Autodesk Fusion 360 part; units mm, degrees
note: some values were not read from the file. Set by a fixed rule: which sketch regions a step uses.
(part 13 of 59)
  spline S70 degree 5 poles (-29.0307, 13.4213) (-29.0307, 13.4213) (-29.0309, 13.4213) (-29.0313, 13.4213) (-29.0318, 13.4213) (-29.0325, 13.4213) (-29.0334, 13.4213) (-29.0344, 13.4214) (-29.0355, 13.4214) (-29.0367, 13.4214) (-29.038, 13.4214) (-29.0394, 13.4214) (-29.0409, 13.4214) (-29.0425, 13.4214) (-29.0443, 13.4214) (-29.0461, 13.4214) (-29.0481, 13.4214) (-29.0501, 13.4214) (-29.0522, 13.4214) (-29.0545, 13.4214) (-29.0568, 13.4214) (-29.0592, 13.4213) (-29.0618, 13.4213) (-29.0644, 13.4212) (-29.0671, 13.4212) (-29.0699, 13.4211) (-29.0728, 13.4211) (-29.0758, 13.421) (-29.0788, 13.4209) (-29.082, 13.4208) (-29.0852, 13.4208) (-29.0886, 13.4206) (-29.092, 13.4205) (-29.0955, 13.4204) (-29.0991, 13.4203) (-29.1028, 13.4201) (-29.1065, 13.42) (-29.1103, 13.4198) (-29.1143, 13.4197) (-29.1183, 13.4195) (-29.1223, 13.4193) (-29.1265, 13.4191) (-29.1307, 13.4189) (-29.135, 13.4186) (-29.1394, 13.4184) (-29.1439, 13.4182) (-29.1484, 13.4179) (-29.153, 13.4176) (-29.1577, 13.4173) (-29.1624, 13.417) (-29.1673, 13.4167) (-29.1722, 13.4164) (-29.1771, 13.4161) (-29.1822, 13.4157) (-29.1873, 13.4153) (-29.1925, 13.415) (-29.1977, 13.4146) (-29.203, 13.4141) (-29.2084, 13.4137) (-29.2139, 13.4133) (-29.2194, 13.4128) (-29.225, 13.4124) (-29.2306, 13.4119) (-29.2363, 13.4114) (-29.2421, 13.4109) (-29.248, 13.4103) (-29.2539, 13.4098) (-29.2599, 13.4092) (-29.2659, 13.4087) (-29.272, 13.4081) (-29.2781, 13.4075) (-29.2844, 13.4068) (-29.2906, 13.4062) (-29.297, 13.4055) (-29.3034, 13.4049) (-29.3099, 13.4042) (-29.3164, 13.4035) (-29.323, 13.4027) (-29.3296, 13.402) (-29.3363, 13.4012) (-29.343, 13.4005) (-29.3498, 13.3997) (-29.3567, 13.3989) (-29.3636, 13.398) (-29.3706, 13.3972) (-29.3777, 13.3963) (-29.3847, 13.3954) (-29.3919, 13.3945) (-29.3991, 13.3936) (-29.4063, 13.3927) (-29.4137, 13.3917) (-29.421, 13.3907) (-29.4284, 13.3897) (-29.4359, 13.3887) (-29.4434, 13.3877) (-29.451, 13.3866) (-29.4586, 13.3856) (-29.4663, 13.3845) (-29.474, 13.3834) (-29.4818, 13.3822) (-29.4896, 13.3811) (-29.4975, 13.3799) (-29.5054, 13.3787) (-29.5134, 13.3775) (-29.5214, 13.3763) (-29.5295, 13.375) (-29.5376, 13.3738) (-29.5458, 13.3725) (-29.554, 13.3712) (-29.5623, 13.3698) (-29.5706, 13.3685) (-29.5789, 13.3671) (-29.5873, 13.3657) (-29.5958, 13.3643) (-29.6043, 13.3629) (-29.6128, 13.3614) (-29.6214, 13.36) (-29.6301, 13.3585) (-29.6388, 13.3569) (-29.6475, 13.3554) (-29.6563, 13.3538) (-29.6651, 13.3523) (-29.6739, 13.3507) (-29.6828, 13.349) (-29.6918, 13.3474) (-29.7008, 13.3457) (-29.7098, 13.344) (-29.7189, 13.3423) (-29.728, 13.3406) (-29.7372, 13.3388) (-29.7464, 13.3371) (-29.7556, 13.3353) (-29.7649, 13.3334) (-29.7742, 13.3316) (-29.7836, 13.3297) (-29.793, 13.3279) (-29.8025, 13.3259) (-29.812, 13.324) (-29.8215, 13.3221) (-29.8311, 13.3201) (-29.8407, 13.3181) (-29.8503, 13.3161) (-29.86, 13.314) (-29.8697, 13.312) (-29.8795, 13.3099) (-29.8893, 13.3078) (-29.8992, 13.3056) (-29.909, 13.3035) (-29.919, 13.3013) (-29.9289, 13.2991) (-29.9389, 13.2969) (-29.949, 13.2946) (-29.959, 13.2923) (-29.9691, 13.29) (-29.9793, 13.2877) (-29.9895, 13.2854) (-29.9997, 13.283) (-30.0099, 13.2806) (-30.0202, 13.2782) (-30.0306, 13.2758) (-30.0409, 13.2733) (-30.0513, 13.2708) (-30.0618, 13.2683) (-30.0722, 13.2658) (-30.0827, 13.2632) (-30.0933, 13.2606) (-30.1038, 13.258) (-30.1145, 13.2554) (-30.1251, 13.2528) (-30.1358, 13.2501) (-30.1465, 13.2474) (-30.1572, 13.2447) (-30.168, 13.2419) (-30.1788, 13.2391) (-30.1897, 13.2364) (-30.2005, 13.2335) (-30.2114, 13.2307) (-30.2224, 13.2278) (-30.2334, 13.2249) (-30.2444, 13.222) (-30.2554, 13.2191) (-30.2665, 13.2161) (-30.2776, 13.2131) (-30.2887, 13.2101) (-30.2999, 13.2071) (-30.3111, 13.204) (-30.3223, 13.2009) (-30.3336, 13.1978) (-30.3448, 13.1947) (-30.3562, 13.1915) (-30.3675, 13.1883) (-30.3789, 13.1851) (-30.3903, 13.1819) (-30.4017, 13.1786) (-30.4132, 13.1753) (-30.4247, 13.172) (-30.4362, 13.1687) (-30.4478, 13.1653) (-30.4594, 13.1619) (-30.471, 13.1585) (-30.4827, 13.1551) (-30.4943, 13.1516) (-30.506, 13.1481) (-30.5178, 13.1446) (-30.5295, 13.1411) (-30.5413, 13.1375) (-30.5531, 13.1339) (-30.565, 13.1303) (-30.5769, 13.1267) (-30.5888, 13.123) (-30.6007, 13.1193) (-30.6126, 13.1156) (-30.6246, 13.1118) (-30.6366, 13.1081) (-30.6487, 13.1043) (-30.6607, 13.1005) (-30.6728, 13.0966) (-30.685, 13.0927) (-30.6971, 13.0889) (-30.7093, 13.0849) (-30.7215, 13.081) (-30.7337, 13.077) (-30.7459, 13.073) (-30.7582, 13.069) (-30.7705, 13.0649) (-30.7828, 13.0609) (-30.7952, 13.0568) (-30.8076, 13.0526) (-30.82, 13.0485) (-30.8324, 13.0443) (-30.8448, 13.0401) (-30.8573, 13.0359) (-30.8698, 13.0316) (-30.8823, 13.0273) (-30.8949, 13.023) (-30.9075, 13.0187) (-30.9201, 13.0143) (-30.9327, 13.0099) (-30.9453, 13.0055) (-30.958, 13.0011) (-30.9707, 12.9966) (-30.9809, 12.993) (-30.9885, 12.9903) (-30.9936, 12.9885) (-30.9962, 12.9876) knots 0 0 0 0 0 0 0.00416667 0.00833333 0.0125 0.01666667 0.02083333 0.025 0.02916667 0.03333333 0.0375 0.04166667 0.04583333 0.05 0.05416667 0.05833333 0.0625 0.06666667 0.07083333 0.075 0.07916667 0.08333333 0.0875 0.09166667 0.09583333 0.1 0.10416667 0.10833333 0.1125 0.11666667 0.12083333 0.125 0.12916667 0.13333333 0.1375 0.14166667 0.14583333 0.15 0.15416667 0.15833333 0.1625 0.16666667 0.17083333 0.175 0.17916667 0.18333333 0.1875 0.19166667 0.19583333 0.2 0.20416667 0.20833333 0.2125 0.21666667 0.22083333 0.225 0.22916667 0.23333333 0.2375 0.24166667 0.24583333 0.25 0.25416667 0.25833333 0.2625 0.26666667 0.27083333 0.275 0.27916667 0.28333333 0.2875 0.29166667 0.29583333 0.3 0.30416667 0.30833333 0.3125 0.31666667 0.32083333 0.325 0.32916667 0.33333333 0.3375 0.34166667 0.34583333 0.35 0.35416667 0.35833333 0.3625 0.36666667 0.37083333 0.375 0.37916667 0.38333333 0.3875 0.39166667 0.39583333 0.4 0.40416667 0.40833333 0.4125 0.41666667 0.42083333 0.425 0.42916667 0.43333333 0.4375 0.44166667 0.44583333 0.45 0.45416667 0.45833333 0.4625 0.46666667 0.47083333 0.475 0.47916667 0.48333333 0.4875 0.49166667 0.49583333 0.5 0.50416667 0.50833333 0.5125 0.51666667 0.52083333 0.525 0.52916667 0.53333333 0.5375 0.54166667 0.54583333 0.55 0.55416667 0.55833333 0.5625 0.56666667 0.57083333 0.575 0.57916667 0.58333333 0.5875 0.59166667 0.59583333 0.6 0.60416667 0.60833333 0.6125 0.61666667 0.62083333 0.625 0.62916667 0.63333333 0.6375 0.64166667 0.64583333 0.65 0.65416667 0.65833333 0.6625 0.66666667 0.67083333 0.675 0.67916667 0.68333333 0.6875 0.69166667 0.69583333 0.7 0.70416667 0.70833333 0.7125 0.71666667 0.72083333 0.725 0.72916667 0.73333333 0.7375 0.74166667 0.74583333 0.75 0.75416667 0.75833333 0.7625 0.76666667 0.77083333 0.775 0.77916667 0.78333333 0.7875 0.79166667 0.79583333 0.8 0.80416667 0.80833333 0.8125 0.81666667 0.82083333 0.825 0.82916667 0.83333333 0.8375 0.84166667 0.84583333 0.85 0.85416667 0.85833333 0.8625 0.86666667 0.87083333 0.875 0.87916667 0.88333333 0.8875 0.89166667 0.89583333 0.9 0.90416667 0.90833333 0.9125 0.91666667 0.92083333 0.925 0.92916667 0.93333333 0.9375 0.94166667 0.94583333 0.95 0.95416667 0.95833333 0.9625 0.96666667 0.97083333 0.975 0.97916667 0.98333333 0.9875 0.99166667 0.99583333 1 1 1 1 1 1
  spline S71 degree 5 poles (15.3132, 37.1806) (15.3132, 37.1807) (15.3133, 37.1809) (15.3135, 37.1812) (15.3138, 37.1816) (15.3142, 37.1822) (15.3146, 37.183) (15.3151, 37.1838) (15.3157, 37.1848) (15.3163, 37.1858) (15.3169, 37.1869) (15.3177, 37.1881) (15.3184, 37.1895) (15.3193, 37.1909) (15.3201, 37.1924) (15.321, 37.194) (15.322, 37.1956) (15.323, 37.1974) (15.3241, 37.1993) (15.3252, 37.2012) (15.3263, 37.2033) (15.3275, 37.2054) (15.3287, 37.2076) (15.33, 37.2099) (15.3313, 37.2122) (15.3327, 37.2147) (15.3341, 37.2172) (15.3355, 37.2198) (15.337, 37.2225) (15.3385, 37.2253) (15.34, 37.2282) (15.3416, 37.2311) (15.3432, 37.2341) (15.3449, 37.2372) (15.3465, 37.2404) (15.3482, 37.2437) (15.35, 37.247) (15.3518, 37.2504) (15.3536, 37.2539) (15.3554, 37.2574) (15.3573, 37.261) (15.3592, 37.2647) (15.3611, 37.2685) (15.3631, 37.2723) (15.3651, 37.2763) (15.3671, 37.2802) (15.3691, 37.2843) (15.3712, 37.2884) (15.3733, 37.2926) (15.3754, 37.2969) (15.3775, 37.3012) (15.3797, 37.3056) (15.3819, 37.3101) (15.3841, 37.3147) (15.3863, 37.3193) (15.3886, 37.3239) (15.3909, 37.3287) (15.3932, 37.3335) (15.3955, 37.3384) (15.3979, 37.3433) (15.4002, 37.3483) (15.4026, 37.3534) (15.405, 37.3585) (15.4075, 37.3637) (15.4099, 37.369) (15.4124, 37.3743) (15.4149, 37.3797) (15.4174, 37.3852) (15.4199, 37.3907) (15.4224, 37.3962) (15.425, 37.4019) (15.4275, 37.4076) (15.4301, 37.4133) (15.4327, 37.4192) (15.4353, 37.425) (15.438, 37.431) (15.4406, 37.437) (15.4433, 37.443) (15.446, 37.4492) (15.4486, 37.4553) (15.4514, 37.4616) (15.4541, 37.4679) (15.4568, 37.4742) (15.4595, 37.4806) (15.4623, 37.4871) (15.4651, 37.4936) (15.4678, 37.5002) (15.4706, 37.5069) (15.4734, 37.5136) (15.4762, 37.5203) (15.4791, 37.5271) (15.4819, 37.534) (15.4848, 37.5409) (15.4876, 37.5479) (15.4905, 37.5549) (15.4933, 37.562) (15.4962, 37.5691) (15.4991, 37.5763) (15.502, 37.5836) (15.5049, 37.5909) (15.5078, 37.5982) (15.5108, 37.6056) (15.5137, 37.6131) (15.5166, 37.6206) (15.5196, 37.6282) (15.5226, 37.6358) (15.5255, 37.6434) (15.5285, 37.6512) (15.5315, 37.6589) (15.5344, 37.6668) (15.5374, 37.6746) (15.5404, 37.6826) (15.5434, 37.6905) (15.5464, 37.6986) (15.5494, 37.7066) (15.5524, 37.7148) (15.5555, 37.7229) (15.5585, 37.7312) (15.5615, 37.7394) (15.5645, 37.7478) (15.5676, 37.7562) (15.5706, 37.7646) (15.5737, 37.7731) (15.5767, 37.7816) (15.5798, 37.7901) (15.5828, 37.7988) (15.5859, 37.8074) (15.5889, 37.8161) (15.592, 37.8249) (15.595, 37.8337) (15.5981, 37.8426) (15.6012, 37.8515) (15.6042, 37.8604) (15.6073, 37.8694) (15.6104, 37.8785) (15.6134, 37.8876) (15.6165, 37.8967) (15.6196, 37.9059) (15.6227, 37.9151) (15.6257, 37.9244) (15.6288, 37.9337) (15.6319, 37.9431) (15.635, 37.9525) (15.638, 37.962) (15.6411, 37.9715) (15.6442, 37.981) (15.6473, 37.9906) (15.6503, 38.0003) (15.6534, 38.0099) (15.6565, 38.0197) (15.6596, 38.0294) (15.6626, 38.0393) (15.6657, 38.0491) (15.6688, 38.059) (15.6718, 38.069) (15.6749, 38.079) (15.6779, 38.089) (15.681, 38.0991) (15.6841, 38.1092) (15.6871, 38.1194) (15.6902, 38.1296) (15.6932, 38.1398) (15.6963, 38.1501) (15.6993, 38.1604) (15.7023, 38.1708) (15.7054, 38.1812) (15.7084, 38.1917) (15.7114, 38.2022) (15.7145, 38.2127) (15.7175, 38.2233) (15.7205, 38.2339) (15.7235, 38.2446) (15.7265, 38.2553) (15.7295, 38.266) (15.7325, 38.2768) (15.7355, 38.2877) (15.7385, 38.2985) (15.7415, 38.3094) (15.7445, 38.3204) (15.7475, 38.3314) (15.7504, 38.3424) (15.7534, 38.3535) (15.7564, 38.3646) (15.7593, 38.3757) (15.7623, 38.3869) (15.7652, 38.3982) (15.7682, 38.4094) (15.7711, 38.4207) (15.774, 38.4321) (15.7769, 38.4435) (15.7798, 38.4549) (15.7828, 38.4663) (15.7857, 38.4778) (15.7886, 38.4894) (15.7914, 38.501) (15.7943, 38.5126) (15.7972, 38.5242) (15.8001, 38.5359) (15.8029, 38.5477) (15.8058, 38.5594) (15.8086, 38.5712) (15.8115, 38.5831) (15.8143, 38.595) (15.8171, 38.6069) (15.8199, 38.6188) (15.8227, 38.6308) (15.8255, 38.6428) (15.8283, 38.6549) (15.8311, 38.667) (15.8339, 38.6792) (15.8367, 38.6913) (15.8394, 38.7035) (15.8422, 38.7158) (15.8449, 38.7281) (15.8477, 38.7404) (15.8504, 38.7528) (15.8531, 38.7651) (15.8558, 38.7776) (15.8585, 38.79) (15.8612, 38.8025) (15.8639, 38.8151) (15.8666, 38.8276) (15.8692, 38.8403) (15.8719, 38.8529) (15.8745, 38.8656) (15.8771, 38.8783) (15.8798, 38.891) (15.8824, 38.9038) (15.885, 38.9166) (15.8876, 38.9295) (15.8902, 38.9424) (15.8927, 38.9553) (15.8953, 38.9682) (15.8979, 38.9812) (15.9004, 38.9943) (15.9029, 39.0073) (15.9055, 39.0204) (15.908, 39.0335) (15.9105, 39.0467) (15.913, 39.0599) (15.9154, 39.0731) (15.9174, 39.0837) (15.9189, 39.0917) (15.9199, 39.097) (15.9204, 39.0997) knots 0 0 0 0 0 0 0.00416667 0.00833333 0.0125 0.01666667 0.02083333 0.025 0.02916667 0.03333333 0.0375 0.04166667 0.04583333 0.05 0.05416667 0.05833333 0.0625 0.06666667 0.07083333 0.075 0.07916667 0.08333333 0.0875 0.09166667 0.09583333 0.1 0.10416667 0.10833333 0.1125 0.11666667 0.12083333 0.125 0.12916667 0.13333333 0.1375 0.14166667 0.14583333 0.15 0.15416667 0.15833333 0.1625 0.16666667 0.17083333 0.175 0.17916667 0.18333333 0.1875 0.19166667 0.19583333 0.2 0.20416667 0.20833333 0.2125 0.21666667 0.22083333 0.225 0.22916667 0.23333333 0.2375 0.24166667 0.24583333 0.25 0.25416667 0.25833333 0.2625 0.26666667 0.27083333 0.275 0.27916667 0.28333333 0.2875 0.29166667 0.29583333 0.3 0.30416667 0.30833333 0.3125 0.31666667 0.32083333 0.325 0.32916667 0.33333333 0.3375 0.34166667 0.34583333 0.35 0.35416667 0.35833333 0.3625 0.36666667 0.37083333 0.375 0.37916667 0.38333333 0.3875 0.39166667 0.39583333 0.4 0.40416667 0.40833333 0.4125 0.41666667 0.42083333 0.425 0.42916667 0.43333333 0.4375 0.44166667 0.44583333 0.45 0.45416667 0.45833333 0.4625 0.46666667 0.47083333 0.475 0.47916667 0.48333333 0.4875 0.49166667 0.49583333 0.5 0.50416667 0.50833333 0.5125 0.51666667 0.52083333 0.525 0.52916667 0.53333333 0.5375 0.54166667 0.54583333 0.55 0.55416667 0.55833333 0.5625 0.56666667 0.57083333 0.575 0.57916667 0.58333333 0.5875 0.59166667 0.59583333 0.6 0.60416667 0.60833333 0.6125 0.61666667 0.62083333 0.625 0.62916667 0.63333333 0.6375 0.64166667 0.64583333 0.65 0.65416667 0.65833333 0.6625 0.66666667 0.67083333 0.675 0.67916667 0.68333333 0.6875 0.69166667 0.69583333 0.7 0.70416667 0.70833333 0.7125 0.71666667 0.72083333 0.725 0.72916667 0.73333333 0.7375 0.74166667 0.74583333 0.75 0.75416667 0.75833333 0.7625 0.76666667 0.77083333 0.775 0.77916667 0.78333333 0.7875 0.79166667 0.79583333 0.8 0.80416667 0.80833333 0.8125 0.81666667 0.82083333 0.825 0.82916667 0.83333333 0.8375 0.84166667 0.84583333 0.85 0.85416667 0.85833333 0.8625 0.86666667 0.87083333 0.875 0.87916667 0.88333333 0.8875 0.89166667 0.89583333 0.9 0.90416667 0.90833333 0.9125 0.91666667 0.92083333 0.925 0.92916667 0.93333333 0.9375 0.94166667 0.94583333 0.95 0.95416667 0.95833333 0.9625 0.96666667 0.97083333 0.975 0.97916667 0.98333333 0.9875 0.99166667 0.99583333 1 1 1 1 1 1
  line L155 (29.0298, 11.5787) -> (29.0307, 11.5787)
  arc A82 (26.6221, 1.6453) -> (27.0473, 2.7529) centre (0, 12.5) ccw
  spline S72 degree 5 poles (28.5878, 17.6346) (28.5879, 17.6347) (28.5881, 17.6347) (28.5884, 17.6348) (28.5889, 17.6349) (28.5896, 17.635) (28.5905, 17.6352) (28.5915, 17.6354) (28.5925, 17.6356) (28.5937, 17.6358) (28.595, 17.6361) (28.5964, 17.6363) (28.5979, 17.6367) (28.5995, 17.637) (28.6012, 17.6374) (28.603, 17.6377) (28.6049, 17.6381) (28.6069, 17.6386) (28.6089, 17.639) (28.6111, 17.6395) (28.6134, 17.64) (28.6158, 17.6406) (28.6182, 17.6411) (28.6208, 17.6417) (28.6234, 17.6423) (28.6262, 17.643) (28.629, 17.6436) (28.6319, 17.6443) (28.6349, 17.645) (28.6379, 17.6458) (28.6411, 17.6465) (28.6443, 17.6473) (28.6477, 17.6481) (28.6511, 17.649) (28.6545, 17.6499) (28.6581, 17.6508) (28.6617, 17.6517) (28.6655, 17.6527) (28.6693, 17.6536) (28.6731, 17.6546) (28.6771, 17.6557) (28.6811, 17.6567) (28.6852, 17.6578) (28.6893, 17.6589) (28.6936, 17.6601) (28.6979, 17.6613) (28.7023, 17.6625) (28.7067, 17.6637) (28.7112, 17.6649) (28.7158, 17.6662) (28.7205, 17.6675) (28.7252, 17.6689) (28.73, 17.6702) (28.7349, 17.6716) (28.7398, 17.673) (28.7448, 17.6745) (28.7498, 17.676) (28.7549, 17.6775) (28.7601, 17.679) (28.7654, 17.6806) (28.7707, 17.6822) (28.776, 17.6838) (28.7815, 17.6854) (28.7869, 17.6871) (28.7925, 17.6888) (28.7981, 17.6905) (28.8038, 17.6923) (28.8095, 17.6941) (28.8153, 17.6959) (28.8211, 17.6978) (28.827, 17.6996) (28.833, 17.7015) (28.839, 17.7035) (28.8451, 17.7054) (28.8512, 17.7074) (28.8573, 17.7094) (28.8636, 17.7115) (28.8699, 17.7136) (28.8762, 17.7157) (28.8826, 17.7178) (28.889, 17.72) (28.8955, 17.7222) (28.9021, 17.7244) (28.9087, 17.7266) (28.9153, 17.7289) (28.922, 17.7312) (28.9288, 17.7336) (28.9356, 17.7359) (28.9424, 17.7383) (28.9493, 17.7408) (28.9563, 17.7432) (28.9633, 17.7457) (28.9703, 17.7482) (28.9774, 17.7508) (28.9846, 17.7533) (28.9918, 17.7559) (28.999, 17.7586) (29.0063, 17.7612) (29.0136, 17.7639) (29.021, 17.7666) (29.0284, 17.7694) (29.0358, 17.7722) (29.0433, 17.775) (29.0509, 17.7778) (29.0585, 17.7807) (29.0661, 17.7836) (29.0738, 17.7865) (29.0815, 17.7895) (29.0893, 17.7925) (29.0971, 17.7955) (29.105, 17.7986) (29.1129, 17.8016) (29.1208, 17.8047) (29.1288, 17.8079) (29.1368, 17.8111) (29.1448, 17.8143) (29.1529, 17.8175) (29.1611, 17.8207) (29.1692, 17.824) (29.1775, 17.8273) (29.1857, 17.8307) (29.194, 17.8341) (29.2023, 17.8375) (29.2107, 17.8409) (29.2191, 17.8444) (29.2276, 17.8479) (29.2361, 17.8514) (29.2446, 17.855) (29.2531, 17.8586) (29.2617, 17.8622) (29.2704, 17.8658) (29.279, 17.8695) (29.2878, 17.8732) (29.2965, 17.877) (29.3053, 17.8807) (29.3141, 17.8846) (29.3229, 17.8884) (29.3318, 17.8922) (29.3407, 17.8961) (29.3497, 17.9001) (29.3587, 17.904) (29.3677, 17.908) (29.3767, 17.912) (29.3858, 17.9161) (29.395, 17.9201) (29.4041, 17.9242) (29.4133, 17.9284) (29.4225, 17.9325) (29.4318, 17.9367) (29.441, 17.941) (29.4504, 17.9452) (29.4597, 17.9495) (29.4691, 17.9538) (29.4785, 17.9582) (29.4879, 17.9625) (29.4974, 17.967) (29.5069, 17.9714) (29.5165, 17.9759) (29.526, 17.9804) (29.5356, 17.9849) (29.5452, 17.9895) (29.5549, 17.994) (29.5646, 17.9987) (29.5743, 18.0033) (29.584, 18.008) (29.5938, 18.0127) (29.6036, 18.0175) (29.6134, 18.0222) (29.6233, 18.027) (29.6332, 18.0319) (29.6431, 18.0367) (29.653, 18.0416) (29.663, 18.0466) (29.673, 18.0515) (29.683, 18.0565) (29.6931, 18.0615) (29.7032, 18.0666) (29.7133, 18.0717) (29.7234, 18.0768) (29.7336, 18.0819) (29.7437, 18.0871) (29.754, 18.0923) (29.7642, 18.0975) (29.7745, 18.1028) (29.7847, 18.1081) (29.7951, 18.1134) (29.8054, 18.1188) (29.8158, 18.1242) (29.8262, 18.1296) (29.8366, 18.135) (29.847, 18.1405) (29.8575, 18.146) (29.868, 18.1515) (29.8785, 18.1571) (29.889, 18.1627) (29.8996, 18.1683) (29.9102, 18.174) (29.9208, 18.1797) (29.9314, 18.1854) (29.9421, 18.1912) (29.9527, 18.197) (29.9634, 18.2028) (29.9742, 18.2086) (29.9849, 18.2145) (29.9957, 18.2204) (30.0065, 18.2263) (30.0173, 18.2323) (30.0281, 18.2383) (30.039, 18.2443) (30.0499, 18.2504) (30.0608, 18.2565) (30.0717, 18.2626) (30.0826, 18.2688) (30.0936, 18.2749) (30.1046, 18.2811) (30.1156, 18.2874) (30.1266, 18.2937) (30.1377, 18.3) (30.1487, 18.3063) (30.1598, 18.3127) (30.1709, 18.3191) (30.1821, 18.3255) (30.1932, 18.3319) (30.2044, 18.3384) (30.2156, 18.3449) (30.2268, 18.3515) (30.238, 18.3581) (30.2492, 18.3647) (30.2605, 18.3713) (30.2718, 18.378) (30.2831, 18.3847) (30.2944, 18.3914) (30.3058, 18.3982) (30.3171, 18.405) (30.3285, 18.4118) (30.3399, 18.4187) (30.3513, 18.4255) (30.3628, 18.4325) (30.3742, 18.4394) (30.3857, 18.4464) (30.3972, 18.4534) (30.4064, 18.459) (30.4133, 18.4633) (30.4179, 18.4661) (30.4202, 18.4675) knots 0 0 0 0 0 0 0.00416667 0.00833333 0.0125 0.01666667 0.02083333 0.025 0.02916667 0.03333333 0.0375 0.04166667 0.04583333 0.05 0.05416667 0.05833333 0.0625 0.06666667 0.07083333 0.075 0.07916667 0.08333333 0.0875 0.09166667 0.09583333 0.1 0.10416667 0.10833333 0.1125 0.11666667 0.12083333 0.125 0.12916667 0.13333333 0.1375 0.14166667 0.14583333 0.15 0.15416667 0.15833333 0.1625 0.16666667 0.17083333 0.175 0.17916667 0.18333333 0.1875 0.19166667 0.19583333 0.2 0.20416667 0.20833333 0.2125 0.21666667 0.22083333 0.225 0.22916667 0.23333333 0.2375 0.24166667 0.24583333 0.25 0.25416667 0.25833333 0.2625 0.26666667 0.27083333 0.275 0.27916667 0.28333333 0.2875 0.29166667 0.29583333 0.3 0.30416667 0.30833333 0.3125 0.31666667 0.32083333 0.325 0.32916667 0.33333333 0.3375 0.34166667 0.34583333 0.35 0.35416667 0.35833333 0.3625 0.36666667 0.37083333 0.375 0.37916667 0.38333333 0.3875 0.39166667 0.39583333 0.4 0.40416667 0.40833333 0.4125 0.41666667 0.42083333 0.425 0.42916667 0.43333333 0.4375 0.44166667 0.44583333 0.45 0.45416667 0.45833333 0.4625 0.46666667 0.47083333 0.475 0.47916667 0.48333333 0.4875 0.49166667 0.49583333 0.5 0.50416667 0.50833333 0.5125 0.51666667 0.52083333 0.525 0.52916667 0.53333333 0.5375 0.54166667 0.54583333 0.55 0.55416667 0.55833333 0.5625 0.56666667 0.57083333 0.575 0.57916667 0.58333333 0.5875 0.59166667 0.59583333 0.6 0.60416667 0.60833333 0.6125 0.61666667 0.62083333 0.625 0.62916667 0.63333333 0.6375 0.64166667 0.64583333 0.65 0.65416667 0.65833333 0.6625 0.66666667 0.67083333 0.675 0.67916667 0.68333333 0.6875 0.69166667 0.69583333 0.7 0.70416667 0.70833333 0.7125 0.71666667 0.72083333 0.725 0.72916667 0.73333333 0.7375 0.74166667 0.74583333 0.75 0.75416667 0.75833333 0.7625 0.76666667 0.77083333 0.775 0.77916667 0.78333333 0.7875 0.79166667 0.79583333 0.8 0.80416667 0.80833333 0.8125 0.81666667 0.82083333 0.825 0.82916667 0.83333333 0.8375 0.84166667 0.84583333 0.85 0.85416667 0.85833333 0.8625 0.86666667 0.87083333 0.875 0.87916667 0.88333333 0.8875 0.89166667 0.89583333 0.9 0.90416667 0.90833333 0.9125 0.91666667 0.92083333 0.925 0.92916667 0.93333333 0.9375 0.94166667 0.94583333 0.95 0.95416667 0.95833333 0.9625 0.96666667 0.97083333 0.975 0.97916667 0.98333333 0.9875 0.99166667 0.99583333 1 1 1 1 1 1
  line L156 (28.9679, 10.3817) -> (28.9671, 10.3818)
  line L157 (2.0967, -16.1734) -> (2.1182, -16.4671)
  arc A83 (28.1181, -0.5527) -> (28.5147, 0.3382) centre (0, 12.5) ccw
  spline S73 degree 5 poles (2.755, 43.3773) (2.7539, 43.3749) (2.7515, 43.37) (2.748, 43.3627) (2.7434, 43.353) (2.7376, 43.3408) (2.7319, 43.3287) (2.7262, 43.3165) (2.7205, 43.3044) (2.7149, 43.2924) (2.7092, 43.2803) (2.7036, 43.2683) (2.6981, 43.2563) (2.6925, 43.2443) (2.687, 43.2323) (2.6815, 43.2204) (2.6761, 43.2085) (2.6707, 43.1966) (2.6653, 43.1847) (2.6599, 43.1728) (2.6545, 43.161) (2.6492, 43.1492) (2.6439, 43.1374) (2.6387, 43.1256) (2.6335, 43.1139) (2.6283, 43.1022) (2.6231, 43.0905) (2.6179, 43.0788) (2.6128, 43.0672) (2.6077, 43.0555) (2.6027, 43.0439) (2.5977, 43.0324) (2.5927, 43.0208) (2.5877, 43.0093) (2.5827, 42.9978) (2.5778, 42.9863) (2.5729, 42.9749) (2.5681, 42.9634) (2.5632, 42.952) (2.5584, 42.9407) (2.5537, 42.9293) (2.5489, 42.918) (2.5442, 42.9067) (2.5395, 42.8954) (2.5348, 42.8841) (2.5302, 42.8729) (2.5256, 42.8617) (2.521, 42.8506) (2.5165, 42.8394) (2.5119, 42.8283) (2.5074, 42.8172) (2.503, 42.8061) (2.4985, 42.7951) (2.4941, 42.7841) (2.4897, 42.7731) (2.4854, 42.7621) (2.481, 42.7512) (2.4767, 42.7403) (2.4725, 42.7294) (2.4682, 42.7186) (2.464, 42.7078) (2.4598, 42.697) (2.4557, 42.6862) (2.4515, 42.6755) (2.4474, 42.6648) (2.4433, 42.6541) (2.4393, 42.6435) (2.4353, 42.6329) (2.4313, 42.6223) (2.4273, 42.6118) (2.4234, 42.6012) (2.4194, 42.5907) (2.4156, 42.5803) (2.4117, 42.5699) (2.4079, 42.5595) (2.4041, 42.5491) (2.4003, 42.5388) (2.3965, 42.5284) (2.3928, 42.5182) (2.3891, 42.5079) (2.3855, 42.4977) (2.3818, 42.4875) (2.3782, 42.4774) (2.3746, 42.4673) (2.3711, 42.4572) (2.3675, 42.4471) (2.364, 42.4371) (2.3606, 42.4271) (2.3571, 42.4172) (2.3537, 42.4073) (2.3503, 42.3974) (2.3469, 42.3875) (2.3436, 42.3777) (2.3403, 42.368) (2.337, 42.3582) (2.3337, 42.3485) (2.3305, 42.3388) (2.3273, 42.3292) (2.3241, 42.3196) (2.321, 42.31) (2.3178, 42.3005) (2.3147, 42.291) (2.3117, 42.2815) (2.3086, 42.2721) (2.3056, 42.2627) (2.3026, 42.2534) (2.2996, 42.2441) (2.2967, 42.2348) (2.2938, 42.2255) (2.2909, 42.2163) (2.288, 42.2072) (2.2852, 42.1981) (2.2824, 42.189) (2.2796, 42.1799) (2.2769, 42.1709) (2.2741, 42.1619) (2.2714, 42.153) (2.2688, 42.1441) (2.2661, 42.1353) (2.2635, 42.1265) (2.2609, 42.1177) (2.2583, 42.109) (2.2558, 42.1003) (2.2533, 42.0917) (2.2508, 42.083) (2.2483, 42.0745) (2.2458, 42.066) (2.2434, 42.0575) (2.241, 42.0491) (2.2387, 42.0407) (2.2363, 42.0323) (2.234, 42.024) (2.2317, 42.0158) (2.2295, 42.0075) (2.2272, 41.9994) (2.225, 41.9912) (2.2228, 41.9832) (2.2207, 41.9751) (2.2185, 41.9671) (2.2164, 41.9592) (2.2143, 41.9513) (2.2123, 41.9434) (2.2102, 41.9356) (2.2082, 41.9279) (2.2062, 41.9202) (2.2043, 41.9125) (2.2023, 41.9049) (2.2004, 41.8973) (2.1985, 41.8898) (2.1967, 41.8823) (2.1948, 41.8749) (2.193, 41.8675) (2.1912, 41.8602) (2.1895, 41.8529) (2.1877, 41.8457) (2.186, 41.8386) (2.1843, 41.8314) (2.1827, 41.8244) (2.181, 41.8174) (2.1794, 41.8104) (2.1778, 41.8035) (2.1762, 41.7967) (2.1747, 41.7899) (2.1731, 41.7831) (2.1716, 41.7764) (2.1702, 41.7698) (2.1687, 41.7632) (2.1673, 41.7567) (2.1659, 41.7502) (2.1645, 41.7438) (2.1631, 41.7374) (2.1618, 41.7311) (2.1605, 41.7249) (2.1592, 41.7187) (2.1579, 41.7126) (2.1567, 41.7065) (2.1554, 41.7005) (2.1542, 41.6946) (2.153, 41.6887) (2.1519, 41.6829) (2.1507, 41.6771) (2.1496, 41.6714) (2.1485, 41.6658) (2.1475, 41.6602) (2.1464, 41.6547) (2.1454, 41.6493) (2.1444, 41.6439) (2.1434, 41.6386) (2.1424, 41.6334) (2.1415, 41.6282) (2.1406, 41.6231) (2.1397, 41.618) (2.1388, 41.6131) (2.138, 41.6081) (2.1371, 41.6033) (2.1363, 41.5985) (2.1355, 41.5938) (2.1347, 41.5892) (2.134, 41.5847) (2.1332, 41.5802) (2.1325, 41.5758) (2.1318, 41.5714) (2.1312, 41.5672) (2.1305, 41.563) (2.1299, 41.5589) (2.1292, 41.5549) (2.1286, 41.5509) (2.1281, 41.547) (2.1275, 41.5432) (2.127, 41.5395) (2.1264, 41.5359) (2.1259, 41.5323) (2.1254, 41.5289) (2.125, 41.5255) (2.1245, 41.5222) (2.1241, 41.5189) (2.1237, 41.5158) (2.1233, 41.5128) (2.1229, 41.5098) (2.1225, 41.5069) (2.1222, 41.5041) (2.1219, 41.5015) (2.1215, 41.4989) (2.1212, 41.4963) (2.121, 41.4939) (2.1207, 41.4916) (2.1204, 41.4894) (2.1202, 41.4873) (2.12, 41.4852) (2.1198, 41.4833) (2.1196, 41.4815) (2.1194, 41.4798) (2.1192, 41.4781) (2.1191, 41.4766) (2.1189, 41.4752) (2.1188, 41.4739) (2.1187, 41.4727) (2.1186, 41.4716) (2.1185, 41.4706) (2.1184, 41.4698) (2.1184, 41.469) (2.1183, 41.4685) (2.1183, 41.4682) (2.1183, 41.468) (2.1183, 41.4679) knots -1 -1 -1 -1 -1 -1 -0.99583333 -0.99166667 -0.9875 -0.98333333 -0.97916667 -0.975 -0.97083333 -0.96666667 -0.9625 -0.95833333 -0.95416667 -0.95 -0.94583333 -0.94166667 -0.9375 -0.93333333 -0.92916667 -0.925 -0.92083333 -0.91666667 -0.9125 -0.90833333 -0.90416667 -0.9 -0.89583333 -0.89166667 -0.8875 -0.88333333 -0.87916667 -0.875 -0.87083333 -0.86666667 -0.8625 -0.85833333 -0.85416667 -0.85 -0.84583333 -0.84166667 -0.8375 -0.83333333 -0.82916667 -0.825 -0.82083333 -0.81666667 -0.8125 -0.80833333 -0.80416667 -0.8 -0.79583333 -0.79166667 -0.7875 -0.78333333 -0.77916667 -0.775 -0.77083333 -0.76666667 -0.7625 -0.75833333 -0.75416667 -0.75 -0.74583333 -0.74166667 -0.7375 -0.73333333 -0.72916667 -0.725 -0.72083333 -0.71666667 -0.7125 -0.70833333 -0.70416667 -0.7 -0.69583333 -0.69166667 -0.6875 -0.68333333 -0.67916667 -0.675 -0.67083333 -0.66666667 -0.6625 -0.65833333 -0.65416667 -0.65 -0.64583333 -0.64166667 -0.6375 -0.63333333 -0.62916667 -0.625 -0.62083333 -0.61666667 -0.6125 -0.60833333 -0.60416667 -0.6 -0.59583333 -0.59166667 -0.5875 -0.58333333 -0.57916667 -0.575 -0.57083333 -0.56666667 -0.5625 -0.55833333 -0.55416667 -0.55 -0.54583333 -0.54166667 -0.5375 -0.53333333 -0.52916667 -0.525 -0.52083333 -0.51666667 -0.5125 -0.50833333 -0.50416667 -0.5 -0.49583333 -0.49166667 -0.4875 -0.48333333 -0.47916667 -0.475 -0.47083333 -0.46666667 -0.4625 -0.45833333 -0.45416667 -0.45 -0.44583333 -0.44166667 -0.4375 -0.43333333 -0.42916667 -0.425 -0.42083333 -0.41666667 -0.4125 -0.40833333 -0.40416667 -0.4 -0.39583333 -0.39166667 -0.3875 -0.38333333 -0.37916667 -0.375 -0.37083333 -0.36666667 -0.3625 -0.35833333 -0.35416667 -0.35 -0.34583333 -0.34166667 -0.3375 -0.33333333 -0.32916667 -0.325 -0.32083333 -0.31666667 -0.3125 -0.30833333 -0.30416667 -0.3 -0.29583333 -0.29166667 -0.2875 -0.28333333 -0.27916667 -0.275 -0.27083333 -0.26666667 -0.2625 -0.25833333 -0.25416667 -0.25 -0.24583333 -0.24166667 -0.2375 -0.23333333 -0.22916667 -0.225 -0.22083333 -0.21666667 -0.2125 -0.20833333 -0.20416667 -0.2 -0.19583333 -0.19166667 -0.1875 -0.18333333 -0.17916667 -0.175 -0.17083333 -0.16666667 -0.1625 -0.15833333 -0.15416667 -0.15 -0.14583333 -0.14166667 -0.1375 -0.13333333 -0.12916667 -0.125 -0.12083333 -0.11666667 -0.1125 -0.10833333 -0.10416667 -0.1 -0.09583333 -0.09166667 -0.0875 -0.08333333 -0.07916667 -0.075 -0.07083333 -0.06666667 -0.0625 -0.05833333 -0.05416667 -0.05 -0.04583333 -0.04166667 -0.0375 -0.03333333 -0.02916667 -0.025 -0.02083333 -0.01666667 -0.0125 -0.00833333 -0.00416667 0 0 0 0 0 0
  spline S74 degree 5 poles (24.6806, -2.8132) (24.6807, -2.8132) (24.6809, -2.8133) (24.6812, -2.8135) (24.6816, -2.8138) (24.6822, -2.8142) (24.683, -2.8146) (24.6838, -2.8151) (24.6848, -2.8157) (24.6858, -2.8163) (24.6869, -2.8169) (24.6881, -2.8177) (24.6895, -2.8184) (24.6909, -2.8193) (24.6924, -2.8201) (24.694, -2.821) (24.6956, -2.822) (24.6974, -2.823) (24.6993, -2.8241) (24.7012, -2.8252) (24.7033, -2.8263) (24.7054, -2.8275) (24.7076, -2.8287) (24.7099, -2.83) (24.7122, -2.8313) (24.7147, -2.8327) (24.7172, -2.8341) (24.7198, -2.8355) (24.7225, -2.837) (24.7253, -2.8385) (24.7282, -2.84) (24.7311, -2.8416) (24.7341, -2.8432) (24.7372, -2.8449) (24.7404, -2.8465) (24.7437, -2.8482) (24.747, -2.85) (24.7504, -2.8518) (24.7539, -2.8536) (24.7574, -2.8554) (24.761, -2.8573) (24.7647, -2.8592) (24.7685, -2.8611) (24.7723, -2.8631) (24.7763, -2.8651) (24.7802, -2.8671) (24.7843, -2.8691) (24.7884, -2.8712) (24.7926, -2.8733) (24.7969, -2.8754) (24.8012, -2.8775) (24.8056, -2.8797) (24.8101, -2.8819) (24.8147, -2.8841) (24.8193, -2.8863) (24.8239, -2.8886) (24.8287, -2.8909) (24.8335, -2.8932) (24.8384, -2.8955) (24.8433, -2.8979) (24.8483, -2.9002) (24.8534, -2.9026) (24.8585, -2.905) (24.8637, -2.9075) (24.869, -2.9099) (24.8743, -2.9124) (24.8797, -2.9149) (24.8852, -2.9174) (24.8907, -2.9199) (24.8962, -2.9224) (24.9019, -2.925) (24.9076, -2.9275) (24.9133, -2.9301) (24.9192, -2.9327) (24.925, -2.9353) (24.931, -2.938) (24.937, -2.9406) (24.943, -2.9433) (24.9492, -2.946) (24.9553, -2.9486) (24.9616, -2.9514) (24.9679, -2.9541) (24.9742, -2.9568) (24.9806, -2.9595) (24.9871, -2.9623) (24.9936, -2.9651) (25.0002, -2.9678) (25.0069, -2.9706) (25.0136, -2.9734) (25.0203, -2.9762) (25.0271, -2.9791) (25.034, -2.9819) (25.0409, -2.9848) (25.0479, -2.9876) (25.0549, -2.9905) (25.062, -2.9933) (25.0691, -2.9962) (25.0763, -2.9991) (25.0836, -3.002) (25.0909, -3.0049) (25.0982, -3.0078) (25.1056, -3.0108) (25.1131, -3.0137) (25.1206, -3.0166) (25.1282, -3.0196) (25.1358, -3.0226) (25.1434, -3.0255) (25.1512, -3.0285) (25.1589, -3.0315) (25.1668, -3.0344) (25.1746, -3.0374) (25.1826, -3.0404) (25.1905, -3.0434) (25.1986, -3.0464) (25.2066, -3.0494) (25.2148, -3.0524) (25.2229, -3.0555) (25.2312, -3.0585) (25.2394, -3.0615) (25.2478, -3.0645) (25.2562, -3.0676) (25.2646, -3.0706) (25.2731, -3.0737) (25.2816, -3.0767) (25.2901, -3.0798) (25.2988, -3.0828) (25.3074, -3.0859) (25.3161, -3.0889) (25.3249, -3.092) (25.3337, -3.095) (25.3426, -3.0981) (25.3515, -3.1012) (25.3604, -3.1042) (25.3694, -3.1073) (25.3785, -3.1104) (25.3876, -3.1134) (25.3967, -3.1165) (25.4059, -3.1196) (25.4151, -3.1227) (25.4244, -3.1257) (25.4337, -3.1288) (25.4431, -3.1319) (25.4525, -3.135) (25.462, -3.138) (25.4715, -3.1411) (25.481, -3.1442) (25.4906, -3.1473) (25.5003, -3.1503) (25.5099, -3.1534) (25.5197, -3.1565) (25.5294, -3.1596) (25.5393, -3.1626) (25.5491, -3.1657) (25.559, -3.1688) (25.569, -3.1718) (25.579, -3.1749) (25.589, -3.1779) (25.5991, -3.181) (25.6092, -3.1841) (25.6194, -3.1871) (25.6296, -3.1902) (25.6398, -3.1932) (25.6501, -3.1963) (25.6604, -3.1993) (25.6708, -3.2023) (25.6812, -3.2054) (25.6917, -3.2084) (25.7022, -3.2114) (25.7127, -3.2145) (25.7233, -3.2175) (25.7339, -3.2205) (25.7446, -3.2235) (25.7553, -3.2265) (25.766, -3.2295) (25.7768, -3.2325) (25.7877, -3.2355) (25.7985, -3.2385) (25.8094, -3.2415) (25.8204, -3.2445) (25.8314, -3.2475) (25.8424, -3.2504) (25.8535, -3.2534) (25.8646, -3.2564) (25.8757, -3.2593) (25.8869, -3.2623) (25.8982, -3.2652) (25.9094, -3.2682) (25.9207, -3.2711) (25.9321, -3.274) (25.9435, -3.2769) (25.9549, -3.2798) (25.9663, -3.2828) (25.9778, -3.2857) (25.9894, -3.2886) (26.001, -3.2914) (26.0126, -3.2943) (26.0242, -3.2972) (26.0359, -3.3001) (26.0477, -3.3029) (26.0594, -3.3058) (26.0712, -3.3086) (26.0831, -3.3115) (26.095, -3.3143) (26.1069, -3.3171) (26.1188, -3.3199) (26.1308, -3.3227) (26.1428, -3.3255) (26.1549, -3.3283) (26.167, -3.3311) (26.1792, -3.3339) (26.1913, -3.3367) (26.2035, -3.3394) (26.2158, -3.3422) (26.2281, -3.3449) (26.2404, -3.3477) (26.2528, -3.3504) (26.2651, -3.3531) (26.2776, -3.3558) (26.29, -3.3585) (26.3025, -3.3612) (26.3151, -3.3639) (26.3276, -3.3666) (26.3403, -3.3692) (26.3529, -3.3719) (26.3656, -3.3745) (26.3783, -3.3771) (26.391, -3.3798) (26.4038, -3.3824) (26.4166, -3.385) (26.4295, -3.3876) (26.4424, -3.3902) (26.4553, -3.3927) (26.4682, -3.3953) (26.4812, -3.3979) (26.4943, -3.4004) (26.5073, -3.4029) (26.5204, -3.4055) (26.5335, -3.408) (26.5467, -3.4105) (26.5599, -3.413) (26.5731, -3.4154) (26.5837, -3.4174) (26.5917, -3.4189) (26.597, -3.4199) (26.5997, -3.4204) knots 0 0 0 0 0 0 0.00416667 0.00833333 0.0125 0.01666667 0.02083333 0.025 0.02916667 0.03333333 0.0375 0.04166667 0.04583333 0.05 0.05416667 0.05833333 0.0625 0.06666667 0.07083333 0.075 0.07916667 0.08333333 0.0875 0.09166667 0.09583333 0.1 0.10416667 0.10833333 0.1125 0.11666667 0.12083333 0.125 0.12916667 0.13333333 0.1375 0.14166667 0.14583333 0.15 0.15416667 0.15833333 0.1625 0.16666667 0.17083333 0.175 0.17916667 0.18333333 0.1875 0.19166667 0.19583333 0.2 0.20416667 0.20833333 0.2125 0.21666667 0.22083333 0.225 0.22916667 0.23333333 0.2375 0.24166667 0.24583333 0.25 0.25416667 0.25833333 0.2625 0.26666667 0.27083333 0.275 0.27916667 0.28333333 0.2875 0.29166667 0.29583333 0.3 0.30416667 0.30833333 0.3125 0.31666667 0.32083333 0.325 0.32916667 0.33333333 0.3375 0.34166667 0.34583333 0.35 0.35416667 0.35833333 0.3625 0.36666667 0.37083333 0.375 0.37916667 0.38333333 0.3875 0.39166667 0.39583333 0.4 0.40416667 0.40833333 0.4125 0.41666667 0.42083333 0.425 0.42916667 0.43333333 0.4375 0.44166667 0.44583333 0.45 0.45416667 0.45833333 0.4625 0.46666667 0.47083333 0.475 0.47916667 0.48333333 0.4875 0.49166667 0.49583333 0.5 0.50416667 0.50833333 0.5125 0.51666667 0.52083333 0.525 0.52916667 0.53333333 0.5375 0.54166667 0.54583333 0.55 0.55416667 0.55833333 0.5625 0.56666667 0.57083333 0.575 0.57916667 0.58333333 0.5875 0.59166667 0.59583333 0.6 0.60416667 0.60833333 0.6125 0.61666667 0.62083333 0.625 0.62916667 0.63333333 0.6375 0.64166667 0.64583333 0.65 0.65416667 0.65833333 0.6625 0.66666667 0.67083333 0.675 0.67916667 0.68333333 0.6875 0.69166667 0.69583333 0.7 0.70416667 0.70833333 0.7125 0.71666667 0.72083333 0.725 0.72916667 0.73333333 0.7375 0.74166667 0.74583333 0.75 0.75416667 0.75833333 0.7625 0.76666667 0.77083333 0.775 0.77916667 0.78333333 0.7875 0.79166667 0.79583333 0.8 0.80416667 0.80833333 0.8125 0.81666667 0.82083333 0.825 0.82916667 0.83333333 0.8375 0.84166667 0.84583333 0.85 0.85416667 0.85833333 0.8625 0.86666667 0.87083333 0.875 0.87916667 0.88333333 0.8875 0.89166667 0.89583333 0.9 0.90416667 0.90833333 0.9125 0.91666667 0.92083333 0.925 0.92916667 0.93333333 0.9375 0.94166667 0.94583333 0.95 0.95416667 0.95833333 0.9625 0.96666667 0.97083333 0.975 0.97916667 0.98333333 0.9875 0.99166667 0.99583333 1 1 1 1 1 1
  spline S75 degree 5 poles (28.5147, 0.3382) (28.5128, 0.34) (28.5089, 0.3438) (28.503, 0.3494) (28.4951, 0.3568) (28.4854, 0.366) (28.4756, 0.3752) (28.4658, 0.3844) (28.4561, 0.3935) (28.4464, 0.4027) (28.4366, 0.4117) (28.4269, 0.4208) (28.4172, 0.4298) (28.4075, 0.4387) (28.3978, 0.4477) (28.3882, 0.4566) (28.3785, 0.4655) (28.3689, 0.4743) (28.3593, 0.4831) (28.3496, 0.4919) (28.34, 0.5006) (28.3305, 0.5093) (28.3209, 0.518) (28.3113, 0.5266) (28.3018, 0.5352) (28.2922, 0.5438) (28.2827, 0.5523) (28.2732, 0.5608) (28.2637, 0.5693) (28.2542, 0.5777) (28.2447, 0.5861) (28.2353, 0.5945) (28.2259, 0.6028) (28.2164, 0.6111) (28.207, 0.6193) (28.1976, 0.6276) (28.1882, 0.6357) (28.1789, 0.6439) (28.1695, 0.652) (28.1602, 0.6601) (28.1509, 0.6682) (28.1416, 0.6762) (28.1323, 0.6842) (28.123, 0.6921) (28.1137, 0.7) (28.1045, 0.7079) (28.0953, 0.7157) (28.0861, 0.7235) (28.0769, 0.7313) (28.0677, 0.7391) (28.0585, 0.7468) (28.0494, 0.7544) (28.0403, 0.7621) (28.0312, 0.7697) (28.0221, 0.7772) (28.013, 0.7847) (28.0039, 0.7922) (27.9949, 0.7997) (27.9859, 0.8071) (27.9769, 0.8145) (27.9679, 0.8219) (27.9589, 0.8292) (27.95, 0.8365) (27.9411, 0.8437) (27.9322, 0.8509) (27.9233, 0.8581) (27.9144, 0.8652) (27.9055, 0.8724) (27.8967, 0.8794) (27.8879, 0.8865) (27.8791, 0.8935) (27.8704, 0.9004) (27.8616, 0.9073) (27.8529, 0.9142) (27.8442, 0.9211) (27.8355, 0.9279) (27.8268, 0.9347) (27.8182, 0.9415) (27.8096, 0.9482) (27.801, 0.9548) (27.7924, 0.9615) (27.7838, 0.9681) (27.7753, 0.9747) (27.7668, 0.9812) (27.7583, 0.9877) (27.7498, 0.9942) (27.7414, 1.0006) (27.733, 1.007) (27.7246, 1.0133) (27.7162, 1.0197) (27.7078, 1.0259) (27.6995, 1.0322) (27.6912, 1.0384) (27.6829, 1.0446) (27.6747, 1.0507) (27.6665, 1.0568) (27.6582, 1.0629) (27.6501, 1.0689) (27.6419, 1.0749) (27.6338, 1.0808) (27.6257, 1.0868) (27.6176, 1.0926) (27.6096, 1.0985) (27.6015, 1.1043) (27.5936, 1.1101) (27.5856, 1.1158) (27.5776, 1.1215) (27.5697, 1.1272) (27.5618, 1.1328) (27.554, 1.1384) (27.5462, 1.1439) (27.5384, 1.1494) (27.5306, 1.1549) (27.5228, 1.1604) (27.5151, 1.1658) (27.5074, 1.1711) (27.4998, 1.1765) (27.4922, 1.1817) (27.4846, 1.187) (27.477, 1.1922) (27.4695, 1.1974) (27.462, 1.2025) (27.4545, 1.2076) (27.447, 1.2127) (27.4396, 1.2177) (27.4323, 1.2227) (27.4249, 1.2277) (27.4176, 1.2326) (27.4103, 1.2375) (27.4031, 1.2423) (27.3958, 1.2471) (27.3887, 1.2519) (27.3815, 1.2566) (27.3744, 1.2613) (27.3673, 1.266) (27.3603, 1.2706) (27.3533, 1.2752) (27.3463, 1.2797) (27.3393, 1.2842) (27.3324, 1.2887) (27.3256, 1.2931) (27.3187, 1.2975) (27.3119, 1.3018) (27.3052, 1.3061) (27.2985, 1.3104) (27.2918, 1.3146) (27.2851, 1.3188) (27.2785, 1.323) (27.272, 1.3271) (27.2654, 1.3312) (27.259, 1.3352) (27.2525, 1.3392) (27.2461, 1.3432) (27.2397, 1.3471) (27.2334, 1.351) (27.2271, 1.3549) (27.2209, 1.3587) (27.2147, 1.3624) (27.2085, 1.3662) (27.2024, 1.3699) (27.1963, 1.3735) (27.1903, 1.3771) (27.1843, 1.3807) (27.1784, 1.3842) (27.1725, 1.3877) (27.1666, 1.3912) (27.1608, 1.3946) (27.155, 1.398) (27.1493, 1.4013) (27.1436, 1.4046) (27.138, 1.4079) (27.1324, 1.4111) (27.1269, 1.4143) (27.1214, 1.4174) (27.116, 1.4205) (27.1106, 1.4236) (27.1053, 1.4266) (27.1, 1.4296) (27.0948, 1.4325) (27.0896, 1.4354) (27.0845, 1.4383) (27.0794, 1.4411) (27.0744, 1.4439) (27.0694, 1.4466) (27.0645, 1.4493) (27.0597, 1.452) (27.0549, 1.4546) (27.0501, 1.4572) (27.0454, 1.4597) (27.0408, 1.4622) (27.0362, 1.4647) (27.0317, 1.4671) (27.0272, 1.4694) (27.0228, 1.4718) (27.0185, 1.4741) (27.0142, 1.4763) (27.01, 1.4785) (27.0058, 1.4807) (27.0017, 1.4828) (26.9977, 1.4849) (26.9937, 1.4869) (26.9898, 1.4889) (26.986, 1.4909) (26.9822, 1.4928) (26.9785, 1.4947) (26.9748, 1.4965) (26.9713, 1.4983) (26.9678, 1.5001) (26.9643, 1.5018) (26.961, 1.5034) (26.9577, 1.5051) (26.9544, 1.5066) (26.9513, 1.5082) (26.9482, 1.5097) (26.9452, 1.5111) (26.9423, 1.5125) (26.9394, 1.5139) (26.9366, 1.5152) (26.9339, 1.5165) (26.9313, 1.5177) (26.9288, 1.5189) (26.9263, 1.5201) (26.924, 1.5212) (26.9217, 1.5222) (26.9195, 1.5232) (26.9173, 1.5242) (26.9153, 1.5251) (26.9134, 1.526) (26.9115, 1.5269) (26.9097, 1.5276) (26.908, 1.5284) (26.9065, 1.5291) (26.905, 1.5298) (26.9036, 1.5304) (26.9023, 1.5309) (26.9011, 1.5315) (26.9, 1.5319) (26.899, 1.5324) (26.8981, 1.5328) (26.8973, 1.5331) (26.8966, 1.5334) (26.8961, 1.5336) (26.8958, 1.5337) (26.8956, 1.5338) (26.8955, 1.5338) knots -1 -1 -1 -1 -1 -1 -0.99583333 -0.99166667 -0.9875 -0.98333333 -0.97916667 -0.975 -0.97083333 -0.96666667 -0.9625 -0.95833333 -0.95416667 -0.95 -0.94583333 -0.94166667 -0.9375 -0.93333333 -0.92916667 -0.925 -0.92083333 -0.91666667 -0.9125 -0.90833333 -0.90416667 -0.9 -0.89583333 -0.89166667 -0.8875 -0.88333333 -0.87916667 -0.875 -0.87083333 -0.86666667 -0.8625 -0.85833333 -0.85416667 -0.85 -0.84583333 -0.84166667 -0.8375 -0.83333333 -0.82916667 -0.825 -0.82083333 -0.81666667 -0.8125 -0.80833333 -0.80416667 -0.8 -0.79583333 -0.79166667 -0.7875 -0.78333333 -0.77916667 -0.775 -0.77083333 -0.76666667 -0.7625 -0.75833333 -0.75416667 -0.75 -0.74583333 -0.74166667 -0.7375 -0.73333333 -0.72916667 -0.725 -0.72083333 -0.71666667 -0.7125 -0.70833333 -0.70416667 -0.7 -0.69583333 -0.69166667 -0.6875 -0.68333333 -0.67916667 -0.675 -0.67083333 -0.66666667 -0.6625 -0.65833333 -0.65416667 -0.65 -0.64583333 -0.64166667 -0.6375 -0.63333333 -0.62916667 -0.625 -0.62083333 -0.61666667 -0.6125 -0.60833333 -0.60416667 -0.6 -0.59583333 -0.59166667 -0.5875 -0.58333333 -0.57916667 -0.575 -0.57083333 -0.56666667 -0.5625 -0.55833333 -0.55416667 -0.55 -0.54583333 -0.54166667 -0.5375 -0.53333333 -0.52916667 -0.525 -0.52083333 -0.51666667 -0.5125 -0.50833333 -0.50416667 -0.5 -0.49583333 -0.49166667 -0.4875 -0.48333333 -0.47916667 -0.475 -0.47083333 -0.46666667 -0.4625 -0.45833333 -0.45416667 -0.45 -0.44583333 -0.44166667 -0.4375 -0.43333333 -0.42916667 -0.425 -0.42083333 -0.41666667 -0.4125 -0.40833333 -0.40416667 -0.4 -0.39583333 -0.39166667 -0.3875 -0.38333333 -0.37916667 -0.375 -0.37083333 -0.36666667 -0.3625 -0.35833333 -0.35416667 -0.35 -0.34583333 -0.34166667 -0.3375 -0.33333333 -0.32916667 -0.325 -0.32083333 -0.31666667 -0.3125 -0.30833333 -0.30416667 -0.3 -0.29583333 -0.29166667 -0.2875 -0.28333333 -0.27916667 -0.275 -0.27083333 -0.26666667 -0.2625 -0.25833333 -0.25416667 -0.25 -0.24583333 -0.24166667 -0.2375 -0.23333333 -0.22916667 -0.225 -0.22083333 -0.21666667 -0.2125 -0.20833333 -0.20416667 -0.2 -0.19583333 -0.19166667 -0.1875 -0.18333333 -0.17916667 -0.175 -0.17083333 -0.16666667 -0.1625 -0.15833333 -0.15416667 -0.15 -0.14583333 -0.14166667 -0.1375 -0.13333333 -0.12916667 -0.125 -0.12083333 -0.11666667 -0.1125 -0.10833333 -0.10416667 -0.1 -0.09583333 -0.09166667 -0.0875 -0.08333333 -0.07916667 -0.075 -0.07083333 -0.06666667 -0.0625 -0.05833333 -0.05416667 -0.05 -0.04583333 -0.04166667 -0.0375 -0.03333333 -0.02916667 -0.025 -0.02083333 -0.01666667 -0.0125 -0.00833333 -0.00416667 0 0 0 0 0 0
  spline S76 degree 5 poles (27.0873, -2.5758) (27.0855, -2.5737) (27.082, -2.5696) (27.0767, -2.5635) (27.0697, -2.5553) (27.061, -2.545) (27.0522, -2.5349) (27.0435, -2.5247) (27.0347, -2.5146) (27.026, -2.5045) (27.0173, -2.4945) (27.0086, -2.4845) (26.9999, -2.4745) (26.9912, -2.4646) (26.9825, -2.4547) (26.9738, -2.4448) (26.9651, -2.435) (26.9565, -2.4252) (26.9478, -2.4154) (26.9392, -2.4057) (26.9305, -2.396) (26.9219, -2.3863) (26.9133, -2.3767) (26.9047, -2.3671) (26.8961, -2.3576) (26.8875, -2.3481) (26.8789, -2.3386) (26.8703, -2.3291) (26.8618, -2.3197) (26.8532, -2.3104) (26.8447, -2.301) (26.8361, -2.2917) (26.8276, -2.2824) (26.8191, -2.2732) (26.8106, -2.264) (26.8021, -2.2549) (26.7937, -2.2457) (26.7852, -2.2366) (26.7767, -2.2276) (26.7683, -2.2186) (26.7599, -2.2096) (26.7515, -2.2006) (26.7431, -2.1917) (26.7347, -2.1829) (26.7263, -2.174) (26.7179, -2.1652) (26.7096, -2.1565) (26.7012, -2.1477) (26.6929, -2.139) (26.6846, -2.1304) (26.6763, -2.1218) (26.668, -2.1132) (26.6597, -2.1046) (26.6514, -2.0961) (26.6432, -2.0877) (26.635, -2.0792) (26.6267, -2.0708) (26.6185, -2.0625) (26.6103, -2.0541) (26.6022, -2.0459) (26.594, -2.0376) (26.5858, -2.0294) (26.5777, -2.0212) (26.5696, -2.0131) (26.5615, -2.005) (26.5534, -1.9969) (26.5453, -1.9889) (26.5373, -1.9809) (26.5292, -1.9729) (26.5212, -1.965) (26.5132, -1.9571) (26.5052, -1.9493) (26.4972, -1.9415) (26.4893, -1.9337) (26.4813, -1.926) (26.4734, -1.9183) (26.4655, -1.9106) (26.4576, -1.903) (26.4497, -1.8954) (26.4419, -1.8879) (26.434, -1.8804) (26.4262, -1.8729) (26.4184, -1.8655) (26.4106, -1.8581) (26.4029, -1.8508) (26.3951, -1.8435) (26.3874, -1.8362) (26.3797, -1.8289) (26.372, -1.8217) (26.3643, -1.8146) (26.3567, -1.8075) (26.3491, -1.8004) (26.3414, -1.7933) (26.3339, -1.7863) (26.3263, -1.7794) (26.3188, -1.7724) (26.3112, -1.7656) (26.3037, -1.7587) (26.2962, -1.7519) (26.2888, -1.7451) (26.2813, -1.7384) (26.2739, -1.7317) (26.2665, -1.725) (26.2592, -1.7184) (26.2518, -1.7119) (26.2445, -1.7053) (26.2372, -1.6988) (26.2299, -1.6924) (26.2227, -1.6859) (26.2154, -1.6796) (26.2082, -1.6732) (26.201, -1.6669) (26.1939, -1.6607) (26.1868, -1.6544) (26.1796, -1.6483) (26.1726, -1.6421) (26.1655, -1.636) (26.1585, -1.63) (26.1515, -1.6239) (26.1445, -1.618) (26.1375, -1.612) (26.1306, -1.6061) (26.1237, -1.6003) (26.1168, -1.5945) (26.11, -1.5887) (26.1032, -1.5829) (26.0964, -1.5772) (26.0896, -1.5716) (26.0829, -1.566) (26.0762, -1.5604) (26.0695, -1.5549) (26.0629, -1.5494) (26.0563, -1.5439) (26.0497, -1.5385) (26.0431, -1.5332) (26.0366, -1.5278) (26.0301, -1.5225) (26.0236, -1.5173) (26.0172, -1.5121) (26.0108, -1.5069) (26.0044, -1.5018) (25.9981, -1.4967) (25.9918, -1.4917) (25.9855, -1.4867) (25.9793, -1.4818) (25.9731, -1.4769) (25.9669, -1.472) (25.9608, -1.4672) (25.9547, -1.4624) (25.9486, -1.4576) (25.9426, -1.4529) (25.9366, -1.4483) (25.9306, -1.4437) (25.9247, -1.4391) (25.9188, -1.4346) (25.913, -1.4301) (25.9072, -1.4257) (25.9014, -1.4213) (25.8957, -1.4169) (25.89, -1.4126) (25.8843, -1.4083) (25.8787, -1.4041) (25.8731, -1.3999) (25.8676, -1.3958) (25.8621, -1.3917) (25.8566, -1.3876) (25.8512, -1.3836) (25.8458, -1.3797) (25.8405, -1.3758) (25.8352, -1.3719) (25.8299, -1.3681) (25.8247, -1.3643) (25.8195, -1.3605) (25.8144, -1.3568) (25.8093, -1.3532) (25.8043, -1.3496) (25.7993, -1.346) (25.7944, -1.3425) (25.7895, -1.339) (25.7847, -1.3356) (25.7799, -1.3322) (25.7751, -1.3289) (25.7704, -1.3256) (25.7658, -1.3224) (25.7612, -1.3192) (25.7566, -1.316) (25.7521, -1.3129) (25.7476, -1.3098) (25.7432, -1.3068) (25.7389, -1.3039) (25.7346, -1.3009) (25.7304, -1.2981) (25.7262, -1.2952) (25.722, -1.2925) (25.718, -1.2897) (25.7139, -1.287) (25.71, -1.2844) (25.706, -1.2818) (25.7022, -1.2793) (25.6984, -1.2768) (25.6947, -1.2743) (25.691, -1.2719) (25.6874, -1.2696) (25.6838, -1.2673) (25.6803, -1.265) (25.6769, -1.2628) (25.6735, -1.2607) (25.6702, -1.2586) (25.667, -1.2565) (25.6638, -1.2545) (25.6607, -1.2526) (25.6577, -1.2506) (25.6547, -1.2488) (25.6518, -1.247) (25.6489, -1.2452) (25.6462, -1.2435) (25.6435, -1.2419) (25.6409, -1.2403) (25.6383, -1.2387) (25.6358, -1.2372) (25.6334, -1.2358) (25.6311, -1.2344) (25.6289, -1.233) (25.6267, -1.2317) (25.6246, -1.2305) (25.6226, -1.2293) (25.6207, -1.2282) (25.6188, -1.2271) (25.6171, -1.2261) (25.6154, -1.2251) (25.6138, -1.2242) (25.6123, -1.2233) (25.6109, -1.2225) (25.6096, -1.2217) (25.6083, -1.221) (25.6072, -1.2204) (25.6061, -1.2198) (25.6052, -1.2193) (25.6043, -1.2188) (25.6036, -1.2184) (25.6029, -1.218) (25.6025, -1.2178) (25.6022, -1.2176) (25.602, -1.2175) (25.6019, -1.2175) knots -1 -1 -1 -1 -1 -1 -0.99583333 -0.99166667 -0.9875 -0.98333333 -0.97916667 -0.975 -0.97083333 -0.96666667 -0.9625 -0.95833333 -0.95416667 -0.95 -0.94583333 -0.94166667 -0.9375 -0.93333333 -0.92916667 -0.925 -0.92083333 -0.91666667 -0.9125 -0.90833333 -0.90416667 -0.9 -0.89583333 -0.89166667 -0.8875 -0.88333333 -0.87916667 -0.875 -0.87083333 -0.86666667 -0.8625 -0.85833333 -0.85416667 -0.85 -0.84583333 -0.84166667 -0.8375 -0.83333333 -0.82916667 -0.825 -0.82083333 -0.81666667 -0.8125 -0.80833333 -0.80416667 -0.8 -0.79583333 -0.79166667 -0.7875 -0.78333333 -0.77916667 -0.775 -0.77083333 -0.76666667 -0.7625 -0.75833333 -0.75416667 -0.75 -0.74583333 -0.74166667 -0.7375 -0.73333333 -0.72916667 -0.725 -0.72083333 -0.71666667 -0.7125 -0.70833333 -0.70416667 -0.7 -0.69583333 -0.69166667 -0.6875 -0.68333333 -0.67916667 -0.675 -0.67083333 -0.66666667 -0.6625 -0.65833333 -0.65416667 -0.65 -0.64583333 -0.64166667 -0.6375 -0.63333333 -0.62916667 -0.625 -0.62083333 -0.61666667 -0.6125 -0.60833333 -0.60416667 -0.6 -0.59583333 -0.59166667 -0.5875 -0.58333333 -0.57916667 -0.575 -0.57083333 -0.56666667 -0.5625 -0.55833333 -0.55416667 -0.55 -0.54583333 -0.54166667 -0.5375 -0.53333333 -0.52916667 -0.525 -0.52083333 -0.51666667 -0.5125 -0.50833333 -0.50416667 -0.5 -0.49583333 -0.49166667 -0.4875 -0.48333333 -0.47916667 -0.475 -0.47083333 -0.46666667 -0.4625 -0.45833333 -0.45416667 -0.45 -0.44583333 -0.44166667 -0.4375 -0.43333333 -0.42916667 -0.425 -0.42083333 -0.41666667 -0.4125 -0.40833333 -0.40416667 -0.4 -0.39583333 -0.39166667 -0.3875 -0.38333333 -0.37916667 -0.375 -0.37083333 -0.36666667 -0.3625 -0.35833333 -0.35416667 -0.35 -0.34583333 -0.34166667 -0.3375 -0.33333333 -0.32916667 -0.325 -0.32083333 -0.31666667 -0.3125 -0.30833333 -0.30416667 -0.3 -0.29583333 -0.29166667 -0.2875 -0.28333333 -0.27916667 -0.275 -0.27083333 -0.26666667 -0.2625 -0.25833333 -0.25416667 -0.25 -0.24583333 -0.24166667 -0.2375 -0.23333333 -0.22916667 -0.225 -0.22083333 -0.21666667 -0.2125 -0.20833333 -0.20416667 -0.2 -0.19583333 -0.19166667 -0.1875 -0.18333333 -0.17916667 -0.175 -0.17083333 -0.16666667 -0.1625 -0.15833333 -0.15416667 -0.15 -0.14583333 -0.14166667 -0.1375 -0.13333333 -0.12916667 -0.125 -0.12083333 -0.11666667 -0.1125 -0.10833333 -0.10416667 -0.1 -0.09583333 -0.09166667 -0.0875 -0.08333333 -0.07916667 -0.075 -0.07083333 -0.06666667 -0.0625 -0.05833333 -0.05416667 -0.05 -0.04583333 -0.04166667 -0.0375 -0.03333333 -0.02916667 -0.025 -0.02083333 -0.01666667 -0.0125 -0.00833333 -0.00416667 0 0 0 0 0 0
  line L158 (-8.0945, -15.3937) -> (-8.0125, -15.1109)
  arc A84 (29.3284, 2.4579) -> (29.6298, 3.3854) centre (0, 12.5) ccw